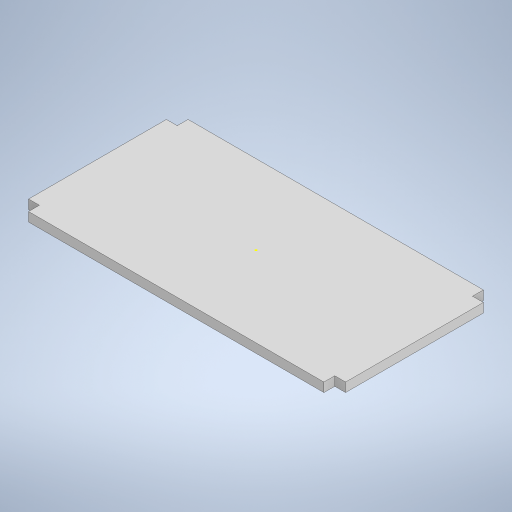
# Autodesk Inventor part: shelf
Saved by Autodesk Inventor 2023 (Build 270158000, 158)
## iProperties
Created: 2023-06-23
Part Number: shelf
Material: Generic
Document SubType Name: Modeling
Designer: incep
Density: 1 g/cm^3
Appearance: Default
Author: incep
Autodesk Inventor part; units mm, degrees
ref_plane "YZ Plane" through (0, 0, 0) normal (1, 0, 0) x (0, 1, 0)
ref_plane "XZ Plane" through (0, 0, 0) normal (0, 1, 0) x (-1, 0, 0)
ref_plane "XY Plane" through (0, 0, 0) normal (0, 0, 1) x (1, 0, 0)
sketch "Sketch1" plane through (0, 0, 0) normal (0, 1, 0) x (-1, 0, 0)
  line L0 (386.4, -194.4) -> (-386.4, -194.4)
  line L1 (-386.4, -194.4) -> (-386.4, 194.4)
  line L2 (-386.4, 194.4) -> (386.4, 194.4)
  line L3 (386.4, 194.4) -> (386.4, -194.4)
  point P0 (0, 0)
  point P1 (-386.4, 0)
  point P2 (0, -194.4)
  dimension "d0" = 772.8
  dimension "d1" = 388.8
  constraints: 8 end point, 2 midpoint, 2 parallel, 1 horizontal, 1 horizontal alignment, 1 perpendicular, 1 vertical alignment
  measures "d0" distance of L1.end L2.end
  measures "d1" distance of L2.end L0.start
extrude "Extrusion1" add sketch "Sketch1" along normal blind 22.225
sketch "Sketch2" plane through (0, 22.225, 0) normal (0, 1, 0) x (1, 0, 0)
  point P0 (0, 0)
sketch "Sketch3" plane through (0, 0, 0) normal (0, -1, 0) x (1, 0, 0)
  line L0 (-387.4, -195.4) -> (387.4, -195.4) construction
  line L1 (387.4, -195.4) -> (387.4, 195.4) construction
  line L2 (387.4, 195.4) -> (-387.4, 195.4) construction
  line L3 (-387.4, 195.4) -> (-387.4, -195.4) construction
  line L4 (-386.4, 194.4) -> (386.4, 194.4) construction
  line L5 (-386.4, -194.4) -> (-386.4, 194.4) construction
  point P0 (0, 0)
  point P1 (-387.4, 0)
  point P2 (0, 195.4)
  dimension "d4" = 1
  dimension "d5" = 1
  constraints: 8 end point, 2 midpoint, 2 parallel, 1 horizontal, 1 horizontal alignment, 1 perpendicular, 1 vertical alignment
  measures "d4" distance between parallel lines of L2 L4
  measures "d5" distance between parallel lines of L5 L3
sketch "Sketch4" plane through (0, 0, 0) normal (0, -1, 0) x (1, 0, 0)
  line L0 (386.4, -194.4) -> (-386.4, -194.4) projected
  line L1 (-386.4, -194.4) -> (-360, -194.4)
  line L2 (-360, -194.4) -> (-360, -168)
  line L3 (-360, -168) -> (-386.4, -168)
  line L4 (-386.4, -168) -> (-386.4, -194.4)
  point P0 (0, 0)
  dimension "d6" = 26.4
  constraints: 8 end point, 2 parallel, 2 perpendicular, 1 horizontal
  measures "d6" distance of L1.end L2.end
extrude "Extrusion2" cut sketch "Sketch4" against normal blind 22.225
mirror "Mirror1" about plane through (0, 0, 0) normal (1, 0, 0) of "Extrusion2"
mirror "Mirror2" about plane through (0, 0, 0) normal (0, 0, 1) of "Extrusion2", "Mirror1"
body "Solid1"
